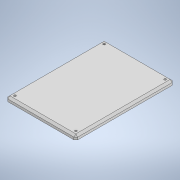
# Autodesk Inventor part: basePlate
Saved by Autodesk Inventor 2022 (Build 260153000, 153)
## iProperties
Created: 2023-11-21
Part Number: basePlate
Material: Generic
Document SubType Name: Modeling
Designer: Timber
Density: 1 g/cm^3
Appearance: Default
Author: Timber
Autodesk Inventor part; units mm, degrees
ref_plane "YZ Plane" through (0, 0, 0) normal (1, 0, 0) x (0, 1, 0)
sketch "Sketch1" plane through (0, 0, 0) normal (0, 1, 0) x (-1, 0, 0)
  line L0 (0, 0) -> (70, 0) construction
  line L1 (70, 0) -> (70, -100) construction
  line L2 (70, -100) -> (0, -100) construction
  line L3 (0, -100) -> (0, 0) construction
  circle A0 centre (2.7, -97.3) radius 1.7 construction
  line L4 (0, -95.6) -> (4.4, -95.6) construction
  line L5 (4.4, -95.6) -> (4.4, -100) construction
  line L6 (72, 2) -> (-2, 2)
  line L7 (-2, 2) -> (-2, -102)
  line L8 (-2, -102) -> (72, -102)
  line L9 (72, -102) -> (72, 2)
  circle A1 centre (2.7, -97.3) radius 2.2
  dimension "d0" = 100
  dimension "d1" = 70
  dimension "d2" = 3.4
  dimension "d3" = 4.4
  dimension "d4" = 4.4
  dimension "d5" = 2
  dimension "d6" = 0.5
  constraints: 20 end point, 4 parallel, 4 perpendicular, 2 centre point, 2 point on line, 2 tangent, 1 horizontal, 3 other
  measures "d0" distance of L0.end L1.end
  measures "d1" distance of L1.end L2.end
  measures "d2" diameter of A0
  measures "d3" distance between parallel lines of L3 L5
  measures "d4" distance between parallel lines of L4 L2
  measures "d5" distance between parallel lines of L0 L6
  measures "d6" radial gap between concentric circles of A0 A1
extrude "Extrusion3" add sketch "Sketch1" along normal blind 4.5 contours L9 L8 L7 L6 | A1
extrude "Extrusion4" cut sketch "Sketch1" along normal blind 2.5 contours A1
sketch "Sketch3" plane through (-2.7, 2.5, -97.3) normal (0, -1, 0) x (1, 0, 0)
  circle A0 centre (0, 0) radius 2.2 projected
  circle A1 centre (0, 0) radius 1.1
  point P0 (2.7, 97.3)
  dimension "d16" = 2.2
  constraints: 1 centre point, 1 coincident
  measures "d16" diameter of A1
extrude "Extrusion5" cut sketch "Sketch3" against normal up to surface (2 mm away) contours A1
ref_plane "Work Plane3" through (2, 0, -50) normal (0, 0, -1) x (-1, 0, 0)
ref_plane "Work Plane4" through (-35, 0, -102) normal (-1, 0, 0) x (0, 0, 1)
mirror "Mirror1" about plane through (-35, 0, -102) normal (-1, 0, 0) of "Extrusion4", "Extrusion5"
mirror "Mirror2" about plane through (2, 0, -50) normal (0, 0, -1) of "Extrusion4", "Extrusion5", "Mirror1"
chamfer "Chamfer1" distance 2 angle 45 8 edges at (-72, 2.25, 2) (2, 2.25, 2) (-72, 2.25, -102) (2, 2.25, -102) (-35, 4.5, -102) (2, 4.5, -50) (-72, 4.5, -50) (-35, 4.5, 2)
body "Solid2"
